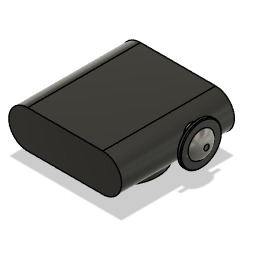
Tête (Autodesk Fusion 360 design; units mm, degrees)
Autodesk Fusion 360 part; units mm, degrees
sketch "Sketch1" plane through (0, 0, 0) normal (0, 0, 1) x (1, 0, 0)
  line L0 (50, 50) -> (0, 50)
  line L1 (0, 50) -> (0, 48)
  arc A0 (50, 0) -> (50, 50) centre (50, 25) ccw
  line L2 (0, 48) -> (48, 48)
  arc A1 (50, 2.0871) -> (48, 48) centre (48, 25) ccw
  arc A2 (-48, 48) -> (-50, 2.0871) centre (-48, 25) ccw
  line L3 (0, 50) -> (0, 48)
  line L4 (-50, 50) -> (0, 50)
  arc A3 (-50, 50) -> (-50, 0) centre (-50, 25) ccw
  line L5 (0, 48) -> (-48, 48)
  line L6 (100, -50) -> (-100, -50)
  line L7 (-100, -50) -> (-100, 100)
  line L8 (-100, 100) -> (100, 100)
  line L9 (100, 100) -> (100, -50)
  line L10 (30.6667, 48) -> (33.3333, 50) construction
  line L11 (-50, 2.0871) -> (-50, 0)
  line L12 (50, 2.0871) -> (50, 0)
  line L13 (-30.6667, 48) -> (-33.3333, 50) construction
  line L14 (-50, 2.0871) -> (50, 2.0871)
  dimension "d1" = 50
  dimension "d2" = 50
  dimension "d8" = 46
  dimension "d9" = 200
  dimension "d10" = 150
  constraint horizontal L0
  constraint vertical L1
  constraint tangent L0 A0
  constraint symmetric A0.start L1 A3.end
  constraint symmetric L0.start L1 L4.start
  constraint symmetric L0.end L1 L3.start
  constraint symmetric L1 A0 A3
  constraint symmetric L1 L2.end A2.start
  constraint symmetric L1 A1 A2
  constraint horizontal L6
  constraint perpendicular L6 L7
  constraint parallel L6 L8
  constraint parallel L7 L9
  constraint vertical L11
  constraint parallel L7 L12
  constraint coincident L2 L10.start
  constraint coincident L5 L13.start
  constraint coincident L0 L10.end
  constraint coincident L4 L13.end
  measures "d1" distance of origin A0.start
  measures "d2" distance of origin L0.end
  measures "d8" diameter of A1
  measures "d9" distance of L7.end L8.end
  measures "d10" distance of L6.end L7.end
extrude "Extrude1" add sketch "Sketch1" along normal blind 146 contours L0 L1 A0 L2 A1 L3 L12 | L1 A2 L3 L4 A3 L5 L11 makes body 1
sketch "Sketch2" plane through (0, 50, 0) normal (0, 1, 0) x (-1, 0, 0)
  line L0 (-50, 0) -> (50, 0)
  line L1 (50, 0) -> (50, 146)
  line L2 (50, 146) -> (-50, 146)
  line L3 (-50, 146) -> (-50, 0)
  line L4 (75, 0) -> (-75, 0)
  line L5 (-75, 0) -> (-75, -2)
  line L6 (-75, -2) -> (75, -2)
  line L7 (75, -2) -> (75, 0)
  line L8 (75, 146) -> (-75, 146)
  line L9 (-75, 146) -> (-75, 148)
  line L10 (-75, 148) -> (75, 148)
  line L11 (75, 148) -> (75, 146)
  dimension "d13" = 150
  dimension "d14" = 2
  dimension "d15" = 150
  dimension "d16" = 2
  constraint horizontal L4
  constraint vertical L5
  constraint horizontal L6
  constraint vertical L7
  constraint horizontal L8
  constraint vertical L9
  constraint horizontal L10
  constraint vertical L11
  measures "d13" distance of L4.start L4.end
  measures "d14" distance of L4.start L6.end
  measures "d15" distance of L8.start L8.end
  measures "d16" distance of L8.start L10.end
extrude "Extrude2" add sketch "Sketch2" against normal blind 70 contours L0 L4 L5 L6 L7 | L2 L8 L9 L10 L11 bodies 1
extrude "Extrude3" cut sketch "Sketch1" along normal blind 150 and the other way blind 50 bodies 1
sketch "Sketch3" plane through (0, 2.0871, 0) normal (0, -1, 0) x (1, 0, 0)
  line L0 (50, 148) -> (-50, 148)
  line L1 (-50, 148) -> (-50, 146)
  line L2 (-50, 146) -> (50, 146)
  line L3 (50, 146) -> (50, 148)
  circle A0 centre (0, 73) radius 48
  circle A1 centre (0, 73) radius 46
  line L4 (-50, 148) -> (50, 148)
  line L5 (50, 148) -> (50, -2)
  line L6 (50, -2) -> (-50, -2)
  line L7 (-50, -2) -> (-50, 148)
  line L8 (-5, 15) -> (5, 15)
  line L9 (5, 15) -> (5, 131)
  line L10 (5, 131) -> (-5, 131)
  line L11 (-5, 131) -> (-5, 15)
  line L12 (-5, 15) -> (5, 131) construction
  line L13 (5, 15) -> (-5, 131) construction
  line L14 (58, 78) -> (-58, 78)
  line L15 (-58, 78) -> (-58, 68)
  line L16 (-58, 68) -> (58, 68)
  line L17 (58, 68) -> (58, 78)
  line L18 (58, 78) -> (-58, 68) construction
  line L19 (-58, 78) -> (58, 68) construction
  circle A2 centre (0, 67) radius 1
  circle A3 centre (4, 73) radius 1
  circle A4 centre (-4, 73) radius 1
  circle A5 centre (0, 79) radius 1
  point P0 (0, 73)
  point P1 (0, 73)
  dimension "d23" = 96
  dimension "d24" = 75
  dimension "d25" = 92
  dimension "d33" = 116
  dimension "d34" = 10
  dimension "d35" = 2
  dimension "d36" = 2
  dimension "d37" = 2
  dimension "d38" = 2
  dimension "d39" = 12
  dimension "d40" = 6
  dimension "d41" = 4
  dimension "d42" = 8
  constraint concentric A0 A1
  constraint horizontal L4
  constraint vertical L5
  constraint horizontal L6
  constraint vertical L7
  constraint coincident L0.end L1.start
  constraint horizontal L8
  constraint perpendicular L8 L9
  constraint parallel L8 L10
  constraint parallel L9 L11
  constraint coincident L12 P1
  constraint coincident L13 P1
  constraint coincident P1 P0
  constraint horizontal L14
  constraint perpendicular L14 L15
  constraint parallel L14 L16
  constraint parallel L15 L17
  constraint coincident L18 P1
  constraint coincident L19 P1
  measures "d23" diameter of A0
  measures "d24" distance of L0 P1
  measures "d25" diameter of A1
  measures "d33" distance of L15.end L16.end
  measures "d34" distance of L14.end L15.end
  measures "d35" diameter of A2
  measures "d36" diameter of A3
  measures "d37" diameter of A4
  measures "d38" diameter of A5
  measures "d39" distance of A2.centre A5.centre
  measures "d40" distance of P1 A2.centre
  measures "d41" distance of P1 A4.centre
  measures "d42" distance of A3.centre A4.centre
extrude "Extrude4" add sketch "Sketch3" along normal blind 2 contours L0 L1 L2 L3 L4 L5 L7 | L2 A0 L5 L7 L9 L10 L11 L14 | A0 L5 L14 L16 | A0 L7 L14 L16 | A0 L5 L6 L7 L8 L9 L11 L16 | A0 L9 L10 L11 | A0 L8 L9 L11 bodies 1
extrude "Extrude5" add sketch "Sketch3" along normal blind 20 contours A0 A1 L9 L14 | A0 A1 L14 L16 | A0 A1 L14 L16 | A0 A1 L11 L14 | A0 A1 L9 L16 | A0 A1 L9 L11 | A0 A1 L11 L16 | A0 A1 L9 L11 bodies 1
sketch "Sketch4" plane through (0, 0, -2) normal (0, 0, -1) x (-1, 0, 0)
  arc A0 (-50, 50) -> (-50, 0) centre (-50, 25) ccw
  line L0 (-50, 0) -> (-50, 0.0871)
  line L1 (-50, 0.0871) -> (50, 0.0871)
  line L2 (50, 0.0871) -> (50, 0)
  arc A1 (50, 0) -> (50, 50) centre (50, 25) ccw
  line L3 (50, 50) -> (-50, 50)
  circle A2 centre (0, 25) radius 17.5
  line L4 (20, 20) -> (-20, 20)
  line L5 (-20, 20) -> (-20, 30)
  line L6 (-20, 30) -> (20, 30)
  line L7 (20, 30) -> (20, 20)
  line L8 (20, 20) -> (-20, 30) construction
  line L9 (-20, 20) -> (20, 30) construction
  line L10 (-6.6445, 5) -> (6.6445, 5)
  line L11 (6.6445, 5) -> (6.6445, 45)
  line L12 (6.6445, 45) -> (-6.6445, 45)
  line L13 (-6.6445, 45) -> (-6.6445, 5)
  line L14 (-6.6445, 5) -> (6.6445, 45) construction
  line L15 (6.6445, 5) -> (-6.6445, 45) construction
  line L16 (13.5, 19) -> (-13.5, 19)
  line L17 (-13.5, 19) -> (-13.5, 31)
  line L18 (-13.5, 31) -> (13.5, 31)
  line L19 (13.5, 31) -> (13.5, 19)
  line L20 (13.5, 19) -> (-13.5, 31) construction
  line L21 (-13.5, 19) -> (13.5, 31) construction
  line L22 (14.5, 18) -> (-14.5, 18)
  line L23 (-14.5, 18) -> (-14.5, 32)
  line L24 (-14.5, 32) -> (14.5, 32)
  line L25 (14.5, 32) -> (14.5, 18)
  line L26 (14.5, 18) -> (-14.5, 32) construction
  line L27 (-14.5, 18) -> (14.5, 32) construction
  point P0 (0, 25)
  point P1 (0, 25)
  point P2 (0, 25)
  point P3 (0, 25)
  dimension "d30" = 35
  dimension "d45" = 40
  dimension "d46" = 10
  dimension "d47" = 40
  dimension "d48" = 27
  dimension "d49" = 12
  dimension "d50" = 29
  dimension "d51" = 14
  constraint horizontal L4
  constraint perpendicular L4 L5
  constraint parallel L4 L6
  constraint parallel L5 L7
  constraint coincident L8 P3
  constraint coincident L9 P3
  constraint coincident P3 P2
  constraint horizontal L10
  constraint perpendicular L10 L11
  constraint parallel L10 L12
  constraint parallel L11 L13
  constraint coincident L14 P3
  constraint coincident L15 P3
  constraint horizontal L16
  constraint perpendicular L16 L17
  constraint parallel L16 L18
  constraint parallel L17 L19
  constraint coincident L20 P3
  constraint coincident L21 P3
  constraint horizontal L22
  constraint perpendicular L22 L23
  constraint parallel L22 L24
  constraint parallel L23 L25
  constraint coincident L26 P3
  constraint coincident L27 P3
  measures "d30" diameter of A2
  measures "d45" distance of L5.end L6.end
  measures "d46" distance of L4.end L5.end
  measures "d47" distance of L10.end L11.end
  measures "d48" distance of L17.end L18.end
  measures "d49" distance of L16.end L17.end
  measures "d50" distance of L23.end L24.end
  measures "d51" distance of L22.end L23.end
extrude "Extrude6" cut sketch "Sketch4" against normal blind 20 contours A2 L4 L6 L25 | A2 L6 L11 L24 L25 | A2 L4 L11 L22 L25 | A2 L11 L13 L24 | L4 L6 L19 L25 | L6 L11 L18 L19 L24 L25 | A2 L11 L13 L22 | L4 L11 L16 L19 L22 L25 | A2 L6 L13 L23 L24 | L11 L13 L18 L24 | L4 L6 L11 L19 | L6 L11 L18 L19 | A2 L4 L13 L22 L23 | L11 L13 L16 L22 | L4 L11 L16 L19 | A2 L4 L6 L23 | L6 L13 L17 L18 L23 L24 | L6 L11 L13 L18 | L4 L6 L11 L13 | L4 L13 L16 L17 L22 L23 | L4 L11 L13 L16 | L4 L6 L17 L23 | L6 L13 L17 L18 | L4 L6 L13 L17 | L4 L13 L16 L17 bodies 1
extrude "Extrude7" add sketch "Sketch3" along normal blind 3 contours A1 L9 L14 L16 | A1 L11 L14 L16 | A1 L9 L11 L14 | L9 L11 L14 L16 | A1 L9 L11 L16 bodies 1
extrude "Extrude8" add sketch "Sketch4" against normal blind 9 contours A2 L4 L6 L7 | A2 L11 L12 L13 | A2 L10 L11 L13 | A2 L4 L5 L6 bodies 1
extrude "Extrude9" add sketch "Sketch4" along normal blind 2 and the other way blind 15 separate body contours L4 L6 L19 L25 | L6 L11 L18 L19 L24 L25 | L4 L11 L16 L19 L22 L25 | L11 L13 L18 L24 | L11 L13 L16 L22 | L6 L13 L17 L18 L23 L24 | L4 L13 L16 L17 L22 L23 | L4 L6 L17 L23 makes body 2
extrude "Extrude10" add sketch "Sketch4" against normal blind 3 from surface at -6 separate body contours A2 L4 L6 L25 | A2 L11 L13 L24 | A2 L11 L13 L22 | A2 L4 L6 L23 makes body 3 at (0, 14.5, 4) makes body 4 at (0, 35.5, 4) makes body 5 at (16.9923, 20.8154, 6) makes body 6 at (-17.4184, 23.3124, 5)
ref_plane "WorkPlane1" through (75, 0, 0) normal (1, 0, 0) x (0, 1, 0)
sketch "Sketch6" plane through (75, 0, 0) normal (1, 0, 0) x (0, 0, -1)
  circle A0 centre (-50, 25) radius 17.5
  circle A1 centre (-50, 25) radius 27.5
  dimension "d62" = 35
  dimension "d63" = 55
  constraint concentric A0 A1
  measures "d62" diameter of A0
  measures "d63" diameter of A1
extrude "Extrude11" add sketch "Sketch6" along normal blind 15 and the other way blind 10 contours A0 bodies 1
extrude "Extrude12" add sketch "Sketch6" along normal blind 5 from surface at 3 bodies 1
fillet "Fillet1" radius 17.5 1 edges at (90, 18.6717, 66.3157) on bodies 1
fillet "Fillet2" radius 1 2 edges at (83, 15.0556, 75.639) (78, 15.0556, 75.639) on bodies 1
